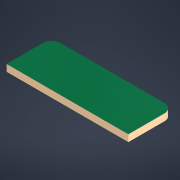
# Autodesk Inventor part: board
Saved by Autodesk Inventor 2021 (Build 250183000, 183)
## iProperties
Created: 2021-01-22
Part Number: board
Material: Generic
Document SubType Name: Modeling
Designer: User
Density: 1 g/cm^3
Appearance: Default
Author: User
Autodesk Inventor part; units mm, degrees
ref_plane "YZ Plane" through (0, 0, 0) normal (1, 0, 0) x (0, 1, 0)
ref_plane "XZ Plane" through (0, 0, 0) normal (0, 1, 0) x (-1, 0, 0)
ref_plane "XY Plane" through (0, 0, 0) normal (0, 0, 1) x (1, 0, 0)
sketch "Sketch1" plane through (0, 0, 0) normal (0, 1, 0) x (-1, 0, 0)
  line L0 (13.5, 5) -> (-13.5, 5)
  line L1 (-13.5, 5) -> (-13.5, -3)
  line L2 (-11.5, -5) -> (11.5, -5)
  line L3 (13.5, -3) -> (13.5, 5)
  line L4 (13.5, 5) -> (-13.5, -5) construction
  line L5 (-13.5, 5) -> (13.5, -5) construction
  arc A0 (11.5, -5) -> (13.5, -3) centre (11.5, -3) ccw
  arc A1 (-13.5, -3) -> (-11.5, -5) centre (-11.5, -3) ccw
  point P0 (0, 0)
  dimension "d0" = 27
  dimension "d1" = 10
  dimension "d2" = 2
  constraints: 12 end point, 4 point on circle, 4 point on line, 4 tangent, 2 centre point, 2 midpoint, 2 parallel, 1 equal radius, 1 horizontal, 1 perpendicular
  measures "d0" distance of L5.end L4.end
  measures "d1" distance of L5.end L0.start
  measures "d2" radius of A0
extrude "Extrusion1" add sketch "Sketch1" along normal blind 1.5
body "Solid1"
